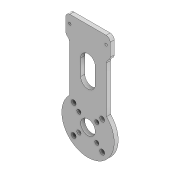
# Autodesk Inventor part: Part2_Camera
Saved by Autodesk Inventor 2021 (Build 250183000, 183)
## iProperties
Created: 2022-06-14
Part Number: Part2_Camera
Material: Generic
Document SubType Name: Modeling
Designer: romanp
Density: 1 g/cm^3
Appearance: Default
Author: romanp
Autodesk Inventor part; units mm, degrees
ref_plane "YZ Plane" through (0, 0, 0) normal (1, 0, 0) x (0, 1, 0)
ref_plane "XZ Plane" through (0, 0, 0) normal (0, 1, 0) x (-1, 0, 0)
ref_plane "XY Plane" through (0, 0, 0) normal (0, 0, 1) x (1, 0, 0)
sketch "Sketch1" plane through (0, 0, 0) normal (0, 0, 1) x (1, 0, 0)
  circle A0 centre (17.6777, -17.6777) radius 3
  circle A1 centre (-17.6777, -17.6777) radius 3
  circle A2 centre (-17.6777, 17.6777) radius 3
  circle A3 centre (17.6777, 17.6777) radius 3
  circle A4 centre (-11.1369, -11.1369) radius 2.5
  circle A5 centre (11.1369, -11.1369) radius 2.5
  circle A6 centre (-11.1369, 11.1369) radius 2.5
  circle A7 centre (11.1369, 11.1369) radius 2.5
  arc A8 (-6.4273, -6.3) -> (-6.4273, 6.3) centre (0, 0) ccw
  arc A9 (-31.8835, -6.3) -> (-31.8835, 6.3) centre (0, 0) ccw
  circle A10 centre (0, 0) radius 32.5
  circle A11 centre (0, 0) radius 9
  line L0 (22.4721, 110) -> (-22.4721, 110)
  line L1 (-27.4721, 105) -> (-27.4721, 90)
  line L2 (-23.0608, 85.5886) -> (-23.0608, 31.884)
  line L3 (23.0603, 31.884) -> (23.0603, 85.5881)
  line L4 (27.4721, 90) -> (27.4721, 105)
  circle A12 centre (22.5, 100) radius 1.5
  circle A13 centre (-22.5, 100) radius 1.5
  circle A14 centre (11.1369, -11.1369) radius 2.5
  circle A15 centre (11.1369, 11.1369) radius 2.5
  circle A16 centre (-11.1369, 11.1369) radius 2.5
  circle A17 centre (-11.1369, -11.1369) radius 2.5
  line L5 (27.4721, 105) -> (27.4721, 110)
  line L6 (27.4721, 110) -> (-27.4721, 110)
  line L7 (-27.4721, 110) -> (-27.4721, 105)
  line L8 (27.4721, 90) -> (27.4721, 85.5881)
  line L9 (27.4721, 85.5881) -> (-27.4721, 85.5881)
  line L10 (-27.4721, 85.5881) -> (-27.4721, 90)
  line L11 (-23.0608, 31.884) -> (-23.0608, 22.9009)
  line L12 (23.0603, 31.884) -> (23.0603, 22.9014)
  point P0 (-31.8835, 6.3)
  point P1 (-23.0608, 85.5881)
  point P2 (-6.4273, 6.3)
  constraints: 26 end point, 18 centre point, 6 point on circle, 2 coincident, 2 concentric, 2 parallel, 2 vertical
extrude "Extrusion1" add sketch "Sketch1" along normal blind 5
fillet "Fillet1" radius 5 6 edges at (-27.4721, 110, 2.5) (27.4721, 110, 2.5) (-27.4721, 85.5881, 2.5) (-23.0608, 85.5881, 2.5) (27.4721, 85.5881, 2.5) (23.0603, 85.5881, 2.5)
sketch "Sketch2" plane through (0, 0, 5) normal (0, 0, 1) x (1, 0, 0)
  circle A0 centre (-22.5, 100) radius 1.5 projected
  arc A1 (9, 70) -> (-9, 70) centre (0, 70) ccw
  line L0 (-9, 70) -> (-9, 50)
  line L1 (9, 70) -> (9, 50)
  line L2 (0, 40) -> (0, 50)
  arc A2 (-9, 50) -> (9, 50) centre (0, 50) ccw
  point P0 (0, 0)
  dimension "d9" = 18
  dimension "d12" = 10
  dimension "d13" = 18
  constraints: 6 end point, 4 point on circle, 2 centre point, 2 tangent, 2 vertical, 1 coincident
  measures "d9" diameter of A1
  measures "d12" distance of L2.start L2.end
  measures "d13" diameter of A2
extrude "Extrusion2" cut sketch "Sketch2" against normal blind 10 contours L1 A2 L0 A1
sketch "Sketch3" plane through (0, 0, 5) normal (0, 0, 1) x (1, 0, 0)
  circle A0 centre (-22.5, 100) radius 1.5 projected
  circle A1 centre (-22.5, 100) radius 1.55
  circle A2 centre (22.5, 100) radius 1.5 projected
  circle A3 centre (22.5, 100) radius 1.55
  circle A4 centre (-17.6777, 17.6777) radius 3 projected
  circle A5 centre (-17.6777, 17.6777) radius 3.05
  circle A6 centre (17.6777, 17.6777) radius 3 projected
  circle A7 centre (17.6777, 17.6777) radius 3.05
  circle A8 centre (17.6777, -17.6777) radius 3 projected
  circle A9 centre (17.6777, -17.6777) radius 3.05
  circle A10 centre (-17.6777, -17.6777) radius 3 projected
  circle A11 centre (-17.6777, -17.6777) radius 3.05
  circle A12 centre (-11.1369, 11.1369) radius 2.5 projected
  circle A13 centre (-11.1369, 11.1369) radius 2.55
  circle A14 centre (11.1369, 11.1369) radius 2.5 projected
  circle A15 centre (11.1369, 11.1369) radius 2.55
  circle A16 centre (11.1369, -11.1369) radius 2.5 projected
  circle A17 centre (11.1369, -11.1369) radius 2.55
  circle A18 centre (-11.1369, -11.1369) radius 2.5 projected
  circle A19 centre (-11.1369, -11.1369) radius 2.55
  point P0 (0, 0)
  dimension "d14" = 3.1
  dimension "d15" = 3.1
  dimension "d16" = 6.1
  dimension "d17" = 6.1
  dimension "d18" = 6.1
  dimension "d19" = 6.1
  dimension "d20" = 5.1
  dimension "d21" = 5.1
  dimension "d22" = 5.1
  dimension "d23" = 5.1
  constraints: 10 centre point, 10 coincident
  measures "d14" diameter of A1
  measures "d15" diameter of A3
  measures "d16" diameter of A5
  measures "d17" diameter of A7
  measures "d18" diameter of A9
  measures "d19" diameter of A11
  measures "d20" diameter of A13
  measures "d21" diameter of A15
  measures "d22" diameter of A17
  measures "d23" diameter of A19
extrude "Extrusion3" cut sketch "Sketch3" against normal blind 10 contours A0 | A1 | A2 | A3 | A4 | A6 | A8 | A9 | A10 | A11 | A12 | A13 | A14 | A15 | A16 | A17 | A18 | A19
body "Solid1"
